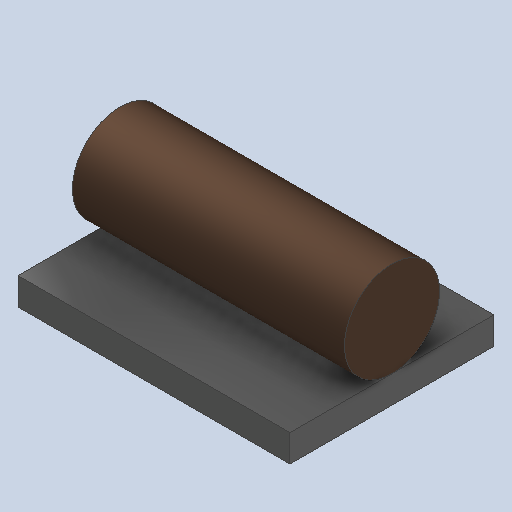
# Autodesk Inventor part: Laser
Saved by Autodesk Inventor 2025.2 (Build 292293000, 293)
## iProperties
Created: 2025-04-08
Part Number: Laser
Material: Generic
Document SubType Name: Modeling
Designer: mirewn
Density: 1 g/cm^3
Appearance: Default
Author: mirewn
Autodesk Inventor part; units mm, degrees
ref_plane "YZ Plane" through (0, 0, 0) normal (1, 0, 0) x (0, 1, 0)
ref_plane "XZ Plane" through (0, 0, 0) normal (0, 1, 0) x (-1, 0, 0)
ref_plane "XY Plane" through (0, 0, 0) normal (0, 0, 1) x (1, 0, 0)
sketch "Sketch1" plane through (0, 0, 0) normal (0, 1, 0) x (-1, 0, 0)
  line L0 (10, 7.5) -> (-10, 7.5)
  line L1 (-10, 7.5) -> (-10, -7.5)
  line L2 (-10, -7.5) -> (10, -7.5)
  line L3 (10, -7.5) -> (10, 7.5)
  line L4 (10, 7.5) -> (-10, -7.5) construction
  line L5 (-10, 7.5) -> (10, -7.5) construction
  point P0 (0, 0)
  dimension "d0" = 20
  dimension "d1" = 15
  constraints: 12 end point, 2 midpoint, 2 parallel, 1 horizontal, 1 perpendicular
  measures "d0" distance of L2.end L1.end
  measures "d1" distance of L1.end L0.end
extrude "Extrusion1" add sketch "Sketch1" along normal blind 9
sketch "Sketch2" plane through (10, 0, 7.5) normal (1, 0, 0) x (0, 0, -1)
  line L0 (0, 0) -> (0, 9) projected
  line L1 (0, 2) -> (15, 2)
  line L2 (15, 0) -> (15, 9) projected
  line L3 (0, 0) -> (15, 0) projected
  line L4 (0, 9) -> (15, 9) construction
  line L5 (7.5, 9) -> (7.5, 2) construction
  circle A0 centre (7.5, 5.5) radius 3.5
  line L6 (0, 2) -> (0, 9)
  line L7 (0, 9) -> (15, 9)
  line L8 (15, 9) -> (15, 2)
  point P0 (7.5, 0)
  point P1 (7.5, 2)
  dimension "d4" = 2
  constraints: 10 end point, 3 midpoint, 2 collinear, 2 point on line, 1 horizontal, 3 other
  measures "d4" distance between parallel lines of L3 L1
extrude "Extrusion2" cut sketch "Sketch2" against normal through all contours L0 L7 A0 L1 | A0 L7 L2 L1
body "Solid1"
